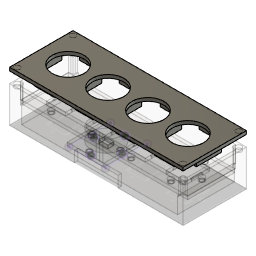
SW Full Enclosure (Autodesk Fusion 360 design; units mm, degrees)
Autodesk Fusion 360 part; units mm, degrees
sketch "Sketch1" plane through (0, 0, 0) normal (0, 1, 0) x (-1, 0, 0) in component "Button"
  arc A0 (78.25, -29) -> (80.25, -27) centre (78.25, -27) ccw
  line L0 (80.25, -27) -> (80.25, 27)
  arc A1 (80.25, 27) -> (78.25, 29) centre (78.25, 27) ccw
  line L1 (78.25, 29) -> (-78.25, 29)
  arc A2 (-78.25, 29) -> (-80.25, 27) centre (-78.25, 27) ccw
  line L2 (-80.25, 27) -> (-80.25, -27)
  arc A3 (-80.25, -27) -> (-78.25, -29) centre (-78.25, -27) ccw
  line L3 (-78.25, -29) -> (78.25, -29)
  circle A4 centre (-18.25, 0) radius 14.75
  circle A5 centre (18.25, 0) radius 14.75
  circle A6 centre (-54.75, 0) radius 14.75
  circle A7 centre (54.75, 0) radius 14.75
  line L4 (35, 19) -> (1.5, 19)
  line L5 (1.5, 19) -> (1.5, -19)
  line L6 (1.5, -19) -> (35, -19)
  line L7 (35, -19) -> (35, 19)
  line L8 (35, 19) -> (1.5, -19) construction
  line L9 (1.5, 19) -> (35, -19) construction
  point P0 (18.25, 0)
  dimension "d261" = 33.5
  dimension "d262" = 38
  dimension "d455" = 18.25
  constraint horizontal L4
  constraint perpendicular L4 L5
  constraint parallel L4 L6
  constraint parallel L5 L7
  constraint coincident L8 P0
  constraint coincident L9 P0
  measures "d261" distance of L5.end L6.end
  measures "d262" distance of L4.end L5.end
  measures "d455" distance of origin A5.centre
extrude "Extrude1" add sketch "Sketch1" along normal blind 3 contours A5 | L4 L5 L6 L7 makes body 1 in component "Button"
sketch "Sketch2" plane through (0, 3, 0) normal (0, 1, 0) x (-1, 0, 0) in component "Button"
  circle A0 centre (31.15, 0) radius 2.6
  line L0 (70, -19) -> (70, 19)
  line L1 (70, 19) -> (38, 19)
  line L2 (38, 19) -> (38, -19)
  line L3 (38, -19) -> (70, -19)
  line L4 (70, 19) -> (38, 19)
  line L5 (70, 19) -> (38, 19)
  line L6 (38, 19) -> (38, -19)
  line L7 (38, -19) -> (70, -19)
  line L8 (70, -19) -> (70, 19)
  line L9 (70, 19) -> (38, 19)
  line L10 (38, 19) -> (38, -19)
  line L11 (38, -19) -> (70, -19)
  circle A1 centre (31.15, 0) radius 2.6
  circle A2 centre (5.35, 0) radius 2.6
  line L12 (35, -19) -> (35, 19)
  line L13 (35, 19) -> (1.5, 19)
  line L14 (1.5, 19) -> (1.5, -19)
  line L15 (1.5, -19) -> (35, -19)
  circle A3 centre (18.25, -15.4) radius 2.6
  circle A4 centre (18.25, 15.4) radius 2.6
  line L16 (26.95, 11.2) -> (9.55, 11.2)
  line L17 (9.55, 11.2) -> (9.55, -11.2)
  line L18 (9.55, -11.2) -> (26.95, -11.2)
  line L19 (26.95, -11.2) -> (26.95, 11.2)
  line L20 (26.95, 11.2) -> (9.55, -11.2) construction
  line L21 (9.55, 11.2) -> (26.95, -11.2) construction
  line L22 (-1.75, 0) -> (-22.5, 0)
  line L23 (18.25, -15.4) -> (18.25, 15.4) construction
  line L24 (31.15, 0) -> (5.35, 0) construction
  point P0 (18.25, 0)
  point P1 (54.75, 0)
  point P2 (18.25, 0)
  point P3 (18.25, 0)
  dimension "d267" = 5.2
  dimension "d456" = 17.4
  dimension "d457" = 22.4
  dimension "d458" = 18.25
  dimension "d459" = 4.2
  dimension "d460" = 4.2
  constraint concentric A0 A1
  constraint equal A1 A4
  constraint equal A0 A2
  constraint equal A3 A4
  constraint horizontal L16
  constraint perpendicular L16 L17
  constraint parallel L16 L18
  constraint parallel L17 L19
  constraint coincident L20 P3
  constraint coincident L21 P3
  constraint coincident P3 L22
  constraint perpendicular L13 L23
  constraint perpendicular L23 L24
  constraint midpoint L23 P3
  constraint coincident P3 P2
  constraint midpoint L24 P3
  constraint coincident A2.centre L24.end
  constraint coincident A3.centre L23.start
  constraint coincident A4.centre L23.end
  constraint coincident A0.centre A1.centre
  constraint equal A2 A3
  measures "d267" diameter of A1
  measures "d456" distance of L17.end L18.end
  measures "d457" distance of L16.end L17.end
  measures "d458" distance of origin P3
  measures "d459" distance of L17 A2.centre
  measures "d460" distance of L18 A3.centre
extrude "Extrude2" cut sketch "Sketch2" along normal blind 2.4 from surface at -3 contours A0 A1 | A2 | A3 | A4 bodies 1 in component "Button"
sketch "Sketch3" plane through (0, 0, 0) normal (0, -1, 0) x (-1, 0, 0) in component "Button"
  circle A0 centre (18.25, -15.4) radius 1.9
  circle A1 centre (18.25, 15.4) radius 1.9
  circle A2 centre (31.15, 0) radius 2.6
  circle A3 centre (5.35, 0) radius 2.6
  circle A4 centre (18.25, 15.4) radius 2.6
  circle A5 centre (18.25, -15.4) radius 2.6
  line L0 (35, -19) -> (35, 19)
  line L1 (35, 19) -> (1.5, 19)
  line L2 (1.5, 19) -> (1.5, -19)
  line L3 (1.5, -19) -> (35, -19)
  circle A6 centre (31.15, 0) radius 1.9
  circle A7 centre (5.35, 0) radius 1.9
  point P0 (18.25, -15.4)
  point P1 (5.35, 0)
  point P2 (31.15, 0)
  point P3 (18.25, 15.4)
  dimension "d272" = 3.8
  dimension "d462" = 3.8
  constraint coincident P0 A0.centre
  constraint coincident P3 A1.centre
  constraint coincident P2 A2.centre
  constraint concentric A3 A7
  constraint equal A6 A7
  constraint equal A0 A7
  measures "d272" diameter of A1
  measures "d462" diameter of A6
extrude "Extrude7" cut sketch "Sketch3" against normal up to surface (3 mm away) contours A0 | A1 | A6 | A7 bodies 1 in component "Button"
sketch "Sketch4" plane through (0, 0, 0) normal (0, 1, 0) x (-1, 0, 0) in component "Button"
  line L0 (35, -19) -> (35, 19)
  line L1 (35, 19) -> (1.5, 19)
  line L2 (1.5, 19) -> (1.5, -19)
  line L3 (1.5, -19) -> (35, -19)
  line L4 (22.5, 2.75) -> (14, 2.75)
  line L5 (14, 2.75) -> (14, -2.75)
  line L6 (14, -2.75) -> (22.5, -2.75)
  line L7 (22.5, -2.75) -> (22.5, 2.75)
  line L8 (22.5, 2.75) -> (14, -2.75) construction
  line L9 (14, 2.75) -> (22.5, -2.75) construction
  line L10 (-1.75, 0) -> (-22.5, 0)
  point P0 (18.25, 0)
  dimension "d290" = 8.5
  dimension "d291" = 5.5
  dimension "d467" = 18.25
  constraint horizontal L4
  constraint perpendicular L4 L5
  constraint parallel L4 L6
  constraint parallel L5 L7
  constraint coincident L8 P0
  constraint coincident L9 P0
  constraint coincident P0 L10
  measures "d290" distance of L5.end L6.end
  measures "d291" distance of L4.end L5.end
  measures "d467" distance of origin P0
extrude "Extrude4" cut sketch "Sketch4" along normal up to surface (3 mm away) contours L4 L5 L6 L7 bodies 1 in component "Button"
sketch "Sketch5" plane through (0, 3, 0) normal (0, 1, 0) x (1, 0, 0) in component "Button"
  line L0 (-35, 19) -> (-35, -19)
  line L1 (-35, -19) -> (-1.5, -19)
  line L2 (-1.5, -19) -> (-1.5, 19)
  line L3 (-1.5, 19) -> (-35, 19)
  circle A0 centre (-18.25, -15.4) radius 1.9
  circle A1 centre (-5.35, 0) radius 1.9
  circle A2 centre (-31.15, 0) radius 1.9
  circle A3 centre (-18.25, 15.4) radius 1.9
  circle A4 centre (-18.25, 0) radius 14
  line L4 (-14, -2.75) -> (-22.5, -2.75)
  line L5 (-22.5, -2.75) -> (-22.5, 2.75)
  line L6 (-22.5, 2.75) -> (-14, 2.75)
  line L7 (-14, 2.75) -> (-14, -2.75)
  circle A5 centre (-18.25, -15.4) radius 1.9
  circle A6 centre (-5.35, 0) radius 1.9
  circle A7 centre (-31.15, 0) radius 1.9
  circle A8 centre (-18.25, 15.4) radius 1.9
  line L8 (-35, 19) -> (-35, -19)
  line L9 (-35, -19) -> (-1.5, -19)
  line L10 (-1.5, -19) -> (-1.5, 19)
  line L11 (-1.5, 19) -> (-35, 19)
  dimension "d465" = 18.25
  dimension "d466" = 28
  measures "d465" distance of origin A4.centre
  measures "d466" diameter of A4
extrude "Extrude5" add sketch "Sketch5" along normal blind 11 separate body contours A0 A4 A5 | A0 A1 A2 A3 A4 A5 A6 A7 A8 | A1 A4 A6 | A2 A4 A7 | A3 A4 A8 | L4 L5 L6 L7 picked at (-18.25, -13.8294) picked at (-5.1201, -0.5681) picked at (-31.2431, 0) picked at (-18.25, 13.8294) makes body 2 in component "Button"
sketch "Sketch6" plane through (0, 0, 0) normal (0, 1, 0) x (1, 0, 0) in component "Button"
  line L0 (-14.1, 2.65) -> (-22.4, 2.65)
  line L1 (-22.4, 2.65) -> (-22.4, -2.65)
  line L2 (-22.4, -2.65) -> (-14.1, -2.65)
  line L3 (-14.1, -2.65) -> (-14.1, 2.65)
  line L4 (-14.1, 2.65) -> (-22.4, -2.65) construction
  line L5 (-22.4, 2.65) -> (-14.1, -2.65) construction
  circle A0 centre (-18.25, 0) radius 14
  point P0 (-18.25, 0)
  dimension "d297" = 8.3
  dimension "d298" = 5.3
  constraint horizontal L0
  constraint perpendicular L0 L1
  constraint parallel L0 L2
  constraint parallel L1 L3
  constraint coincident L4 P0
  constraint coincident L5 P0
  constraint coincident P0 A0.centre
  measures "d297" distance of L1.end L2.end
  measures "d298" distance of L0.end L1.end
extrude "Extrude6" add sketch "Sketch6" along normal blind 7 contours L0 L1 L2 L3 bodies 2 in component "Button"
move_body "Move1" bodies 1 2 to x (1, 0, 0) y (0, 1, 0) z (0, 0, 1) at (-0.7, 0, 0) in component "Button"
move_body "Move2" bodies 2 1 to x (1, 0, 0) y (0, 1, 0) z (0, 0, 1) at (-0.9, 0, 0) in component "Button"
sketch "Sketch1 (2)" plane through (0, 0, 0) normal (0, 1, 0) x (1, 0, 0) in component "Button Base (1)"
  line L0 (76.05, -21.5) -> (0, -21.5)
  line L1 (0, -21.5) -> (0, 21.5)
  line L2 (0, 21.5) -> (76.05, 21.5)
  line L3 (76.05, 21.5) -> (76.05, -21.5)
  line L4 (76.05, -21.5) -> (0, 21.5) construction
  line L5 (0, -21.5) -> (76.05, 21.5) construction
  line L6 (1.75, 0) -> (22.5, 0)
  point P0 (38.025, 0)
  dimension "d337" = 76.05
  dimension "d338" = 43
  constraint horizontal L0
  constraint perpendicular L0 L1
  constraint parallel L0 L2
  constraint parallel L1 L3
  constraint coincident L4 P0
  constraint coincident L5 P0
  constraint coincident P0 L6
  constraint coincident origin L1
  measures "d337" distance of L1.end L2.end
  measures "d338" distance of L0.start L2.end
extrude "Extrude1'" add sketch "Sketch1 (2)" along normal blind 3 separate body makes body 3 in component "Button Base (1)"
sketch "Sketch2 (2)" plane through (0, 3, 0) normal (0, 1, 0) x (-1, 0, 0) in component "Button Base (1)"
  line L0 (-76.05, -21.5) -> (0, -21.5)
  line L1 (0, -21.5) -> (0, 21.5)
  line L2 (0, 21.5) -> (-76.05, 21.5)
  line L3 (-76.05, 21.5) -> (-76.05, -21.5)
  line L4 (-9.55, -11.2) -> (-26.95, -11.2)
  line L5 (-26.95, -11.2) -> (-26.95, 11.2)
  line L6 (-26.95, 11.2) -> (-9.55, 11.2)
  line L7 (-9.55, 11.2) -> (-9.55, -11.2)
  line L8 (-9.55, -11.2) -> (-26.95, 11.2) construction
  line L9 (-26.95, -11.2) -> (-9.55, 11.2) construction
  line L10 (-1.75, 0) -> (-22.5, 0)
  point P0 (-18.25, 0)
  dimension "d341" = 17.4
  dimension "d342" = 22.4
  dimension "d343" = 18.25
  constraint horizontal L4
  constraint perpendicular L4 L5
  constraint parallel L4 L6
  constraint parallel L5 L7
  constraint coincident L8 P0
  constraint coincident L9 P0
  constraint coincident P0 L10
  measures "d341" distance of L5.end L6.end
  measures "d342" distance of L4.end L5.end
  measures "d343" distance of origin P0
extrude "Extrude2'" cut sketch "Sketch2 (2)" against normal up to surface (3 mm away) contours L4 L5 L6 L7 bodies 3 in component "Button Base (1)"
sketch "Sketch3 (2)" plane through (0, 3, 0) normal (0, 1, 0) x (-1, 0, 0) in component "Button Base (1)"
  line L0 (-9.55, 11.2) -> (-9.55, -11.2)
  line L1 (-9.55, -11.2) -> (-26.95, -11.2)
  line L2 (-26.95, -11.2) -> (-26.95, 11.2)
  line L3 (-26.95, 11.2) -> (-9.55, 11.2)
  line L4 (-76.05, -21.5) -> (0, -21.5)
  line L5 (0, -21.5) -> (0, 21.5)
  line L6 (0, 21.5) -> (-76.05, 21.5)
  line L7 (-76.05, 21.5) -> (-76.05, -21.5)
  circle A0 centre (-5.35, 0) radius 2.6
  circle A1 centre (-18.25, -15.4) radius 2.6
  circle A2 centre (-31.15, 0) radius 2.6
  circle A3 centre (-18.25, 15.4) radius 2.6
  line L8 (-18.25, 15.4) -> (-18.25, -15.4) construction
  line L9 (-1.75, 0) -> (-22.5, 0)
  point P0 (-18.25, -11.2)
  dimension "d346" = 5.2
  dimension "d347" = 4.2
  dimension "d348" = 4.2
  dimension "d349" = 4.2
  dimension "d350" = 4.2
  constraint equal A1 A2
  constraint equal A2 A3
  constraint equal A0 A3
  constraint midpoint L1 P0
  constraint perpendicular L1 L8
  constraint coincident A3.centre L8
  constraint coincident A3.centre L8.start
  constraint coincident P0 L8
  constraint coincident A1.centre L8
  constraint coincident A1.centre L8.end
  constraint coincident A2.centre L9
  constraint coincident A0.centre L9
  measures "d346" diameter of A1
  measures "d347" distance of L3 A3.centre
  measures "d348" distance of L1 A1.centre
  measures "d349" distance of L0 A0.centre
  measures "d350" distance of L2 A2.centre
extrude "Extrude3" cut sketch "Sketch3 (2)" against normal blind 2.4 contours A0 L9 | A0 L9 | A1 | A2 | A3 bodies 3 in component "Button Base (1)"
sketch "Sketch4 (2)" plane through (0, 3, 0) normal (0, 1, 0) x (-1, 0, 0) in component "Button Base (1)"
  circle A0 centre (-18.25, -15.4) radius 2.6
  circle A1 centre (-31.15, 0) radius 2.6
  circle A2 centre (-5.35, 0) radius 2.6
  circle A3 centre (-18.25, 15.4) radius 2.6
  line L0 (-9.55, 11.2) -> (-9.55, -11.2)
  line L1 (-9.55, -11.2) -> (-26.95, -11.2)
  line L2 (-26.95, -11.2) -> (-26.95, 11.2)
  line L3 (-26.95, 11.2) -> (-9.55, 11.2)
  line L4 (-76.05, -21.5) -> (0, -21.5)
  line L5 (0, -21.5) -> (0, 21.5)
  line L6 (0, 21.5) -> (-76.05, 21.5)
  line L7 (-76.05, 21.5) -> (-76.05, -21.5)
  circle A4 centre (-18.25, -15.4) radius 1.9
  circle A5 centre (-31.15, 0) radius 1.9
  circle A6 centre (-18.25, 15.4) radius 1.9
  circle A7 centre (-5.35, 0) radius 1.9
  dimension "d353" = 3.8
  constraint concentric A0 A4
  constraint concentric A1 A5
  constraint concentric A3 A6
  constraint concentric A2 A7
  constraint equal A4 A7
  constraint equal A5 A6
  constraint equal A6 A7
  measures "d353" diameter of A7
extrude "Extrude4'" cut sketch "Sketch4 (2)" against normal up to surface (3 mm away) contours A4 | A5 | A6 | A7 bodies 3 in component "Button Base (1)"
sketch "Sketch5 (2)" plane through (0, 0, 21.5) normal (0, 0, 1) x (1, 0, 0) in component "Button Base (1)"
  line L0 (0, 0) -> (76.05, 0)
  line L1 (76.05, 0) -> (76.05, 3)
  line L2 (76.05, 3) -> (0, 3)
  line L3 (0, 3) -> (0, 0)
  line L4 (18.25, 5) -> (18.25, -2) construction
  line L5 (26.95, 0) -> (9.55, 0) construction
  line L6 (9.55, 0) -> (9.55, 3)
  line L7 (9.55, 3) -> (26.95, 3) construction
  line L8 (26.95, 3) -> (26.95, 0) construction
  line L9 (26.95, 0) -> (9.55, 3) construction
  line L10 (9.55, 0) -> (26.95, 3) construction
  line L11 (9.55, 0) -> (11.05, 1.5)
  line L12 (9.55, 0) -> (12.4248, 0) construction
  line L13 (9.55, 3) -> (9.55, 1.5) construction
  line L14 (9.55, 1.5) -> (11.05, 1.5)
  line L15 (9.55, 1.5) -> (9.55, 0) construction
  line L16 (26.95, 0) -> (26.95, 1.5)
  line L17 (26.95, 1.5) -> (25.45, 1.5)
  line L18 (25.45, 1.5) -> (26.95, 0)
  point P0 (18.25, 1.5)
  dimension "d358" = 18.25
  dimension "d359" = 17.4
  dimension "d360" = 3
  dimension "d361" = 45
  dimension "d362" = 1.5
  dimension "d363" = 1.5
  dimension "d364" = 1.5
  dimension "d365" = 1.5
  constraint vertical L4
  constraint horizontal L5
  constraint perpendicular L5 L6
  constraint parallel L5 L7
  constraint parallel L6 L8
  constraint coincident L9 P0
  constraint coincident L10 P0
  constraint midpoint L4 P0
  constraint horizontal L12
  constraint coincident L6 L13.end
  constraint perpendicular L6 L14
  constraint coincident L11.end L14.end
  constraint perpendicular L5 L16
  constraint perpendicular L8 L17
  measures "d358" distance of L0.start L4
  measures "d359" distance of L6.end L7.end
  measures "d360" distance of L5.end L6.end
  measures "d361" angle of L11 L12
  measures "d362" distance of L6.end L13.end
  measures "d363" distance of L0 P0
  measures "d364" distance of L5.start L16.end
  measures "d365" distance of L16.end L17.end
extrude "Extrude5'" add sketch "Sketch5 (2)" along normal mid plane 10 from surface at -21.5 contours L16 L17 L18 | L6 L11 L14 bodies 3 in component "Button Base (1)"
pattern_path "PathPattern1" count 2 spacing 36.5 from (0, 3, -21.5) along 1 edges at (38.025, 3, -21.5) of "Extrude2'", "Extrude3", "Extrude4'", "Extrude5'" on bodies 3 in component "Button Base (1)"
mirror "Mirror1" about plane through (0, 0, 0) normal (1, 0, 0) of bodies 3 makes body 4 in component "Button Base (1)"
combine "Combine1" operation add target body 3 tool bodies 4 in component "Button Base (1)"
sketch "Sketch1 (3)" plane through (0, 0, 0) normal (0, 1, 0) x (1, 0, 0) in component "Button Box (1)"
  line L0 (79.25, -29) -> (0, -29)
  line L1 (0, -29) -> (0, 29)
  line L2 (0, 29) -> (79.25, 29)
  line L3 (79.25, 29) -> (79.25, -29)
  line L4 (79.25, -29) -> (0, 29) construction
  line L5 (0, -29) -> (79.25, 29) construction
  line L6 (1.75, 0) -> (22.5, 0)
  point P0 (39.625, 0)
  dimension "d372" = 79.25
  dimension "d379" = 58
  constraint horizontal L0
  constraint perpendicular L0 L1
  constraint parallel L0 L2
  constraint parallel L1 L3
  constraint coincident L4 P0
  constraint coincident L5 P0
  constraint coincident P0 L6
  constraint coincident origin L1
  measures "d372" distance of L1.end L2.end
  measures "d379" distance of L0.start L2.end
extrude "Extrude1''" add sketch "Sketch1 (3)" along normal blind 33 separate body makes body 5 in component "Button Box (1)"
shell "Shell1" thickness 3 removed faces 1 at (52.8333, 33, 9.6667) on bodies 5 in component "Button Box (1)"
sketch "Sketch2 (3)" plane through (0, 33, 0) normal (0, 1, 0) x (-1, 0, 0) in component "Button Box (1)"
  line L0 (-76.25, -26) -> (-76.25, 26)
  line L1 (-76.25, 26) -> (-3, 26)
  line L2 (-3, 26) -> (-3, -26)
  line L3 (-3, -26) -> (-76.25, -26)
  line L4 (-79.25, -29) -> (0, -29)
  line L5 (0, -29) -> (0, 29)
  line L6 (0, 29) -> (-79.25, 29)
  line L7 (-79.25, 29) -> (-79.25, -29)
  line L8 (-76.25, 26) -> (-71.25, 26)
  line L9 (-71.25, 26) -> (-71.25, -26)
  line L10 (-71.25, -26) -> (-76.25, -26)
  line L11 (-76.25, -26) -> (-76.25, 26)
  line L12 (-76.25, 26) -> (-71.25, -26) construction
  line L13 (-71.25, 26) -> (-76.25, -26) construction
  point P0 (-73.75, 0)
  dimension "d378" = 52
  dimension "d380" = 5
  dimension "d382" = 73.75
  constraint horizontal L8
  constraint perpendicular L8 L9
  constraint parallel L8 L10
  constraint parallel L9 L11
  constraint coincident L1 L0.end
  constraint coincident L12 P0
  constraint coincident L13 P0
  measures "d378" distance of L0.end L0.start
  measures "d380" distance of L9.end L0.start
  measures "d382" distance of origin P0
extrude "Extrude2''" add sketch "Sketch2 (3)" along normal blind 18 from surface at -33 contours L0 L1 L3 L8 L9 L10 L11 bodies 5 in component "Button Box (1)"
sketch "Sketch3 (3)" plane through (0, 33, 0) normal (0, 1, 0) x (-1, 0, 0) in component "Button Box (1)"
  line L0 (-76.25, -26) -> (-76.25, 26)
  line L1 (-76.25, 26) -> (-3, 26)
  line L2 (-3, 26) -> (-3, -26)
  line L3 (-3, -26) -> (-76.25, -26)
  line L4 (-79.25, -29) -> (0, -29)
  line L5 (0, -29) -> (0, 29)
  line L6 (0, 29) -> (-79.25, 29)
  line L7 (-79.25, 29) -> (-79.25, -29)
  line L8 (-79.25, -29) -> (-72.25, -29)
  line L9 (-72.25, -29) -> (-72.25, -22)
  line L10 (-72.25, -22) -> (-79.25, -22)
  line L11 (-79.25, -22) -> (-79.25, -29)
  line L12 (-79.25, 29) -> (-72.25, 29)
  line L13 (-72.25, 29) -> (-72.25, 22)
  line L14 (-72.25, 22) -> (-79.25, 22)
  line L15 (-79.25, 22) -> (-79.25, 29)
  dimension "d386" = 7
  dimension "d387" = 7
  dimension "d388" = 7
  dimension "d389" = 7
  constraint horizontal L8
  constraint vertical L9
  constraint horizontal L10
  constraint vertical L11
  constraint coincident L4.start L7.end
  constraint horizontal L12
  constraint vertical L13
  constraint horizontal L14
  constraint vertical L15
  constraint coincident L6.end L7.start
  measures "d386" distance of L4.start L8.end
  measures "d387" distance of L4.start L10.end
  measures "d388" distance of L6.end L12.end
  measures "d389" distance of L6.end L14.end
extrude "Extrude3'" add sketch "Sketch3 (3)" along normal up to near side of body 5 contours L0 L3 L9 L10 | L0 L1 L13 L14 bodies 5 in component "Button Box (1)"
sketch "Sketch4 (3)" plane through (0, 33, 0) normal (0, 1, 0) x (-1, 0, 0) in component "Button Box (1)"
  line L0 (-76.25, -22) -> (-76.25, 22)
  line L1 (-76.25, 22) -> (-72.25, 22)
  line L2 (-72.25, 22) -> (-72.25, 26)
  line L3 (-72.25, 26) -> (-3, 26)
  line L4 (-3, 26) -> (-3, -26)
  line L5 (-3, -26) -> (-72.25, -26)
  line L6 (-72.25, -26) -> (-72.25, -22)
  line L7 (-72.25, -22) -> (-76.25, -22)
  line L8 (-79.25, -29) -> (0, -29)
  line L9 (0, -29) -> (0, 29)
  line L10 (0, 29) -> (-79.25, 29)
  line L11 (-79.25, 29) -> (-79.25, -29)
  circle A0 centre (-75.75, 25.5) radius 2.6
  circle A1 centre (-75.75, -25.5) radius 2.6
  dimension "d393" = 3.5
  dimension "d394" = 3.5
  dimension "d397" = 3.5
  dimension "d398" = 3.5
  dimension "d399" = 5.2
  constraint equal A0 A1
  measures "d393" distance of L11 A0.centre
  measures "d394" distance of L10 A0.centre
  measures "d397" distance of L8 A1.centre
  measures "d398" distance of L11 A1.centre
  measures "d399" diameter of A1
extrude "Extrude4''" cut sketch "Sketch4 (3)" against normal blind 2.4 contours A0 | A1 bodies 5 in component "Button Box (1)"
fillet "Fillet1" radius 2 2 edges at (72.25, 25.5, 22) (72.25, 25.5, -22) on bodies 5 in component "Button Box (1)"
sketch "Sketch5 (3)" plane through (0, 33, 0) normal (0, 1, 0) x (-1, 0, 0) in component "Button Box (1)"
  arc A0 (-72.25, -24) -> (-74.25, -22) centre (-74.25, -24) ccw
  line L0 (-74.25, -22) -> (-76.25, -22)
  line L1 (-76.25, -22) -> (-76.25, 22)
  line L2 (-76.25, 22) -> (-74.25, 22)
  arc A1 (-74.25, 22) -> (-72.25, 24) centre (-74.25, 24) ccw
  line L3 (-72.25, 24) -> (-72.25, 26)
  line L4 (-72.25, 26) -> (-3, 26)
  line L5 (-3, 26) -> (-3, -26)
  line L6 (-3, -26) -> (-72.25, -26)
  line L7 (-72.25, -26) -> (-72.25, -24)
  circle A2 centre (-75.75, -25.5) radius 2.6
  circle A3 centre (-75.75, 25.5) radius 2.6
  line L8 (-79.25, -29) -> (0, -29)
  line L9 (0, -29) -> (0, 29)
  line L10 (0, 29) -> (-79.25, 29)
  line L11 (-79.25, 29) -> (-79.25, -29)
  line L12 (-3, -26) -> (0, -26)
  line L13 (0, 26) -> (-3, 26)
  constraint coincident L5.end L6.start
  constraint coincident L9 L12.end
  constraint perpendicular L9 L12
  constraint coincident L9 L13.start
  constraint coincident L4.end L5.start
  constraint perpendicular L5 L13
extrude "Extrude5''" cut sketch "Sketch5 (3)" against normal up to surface (30 mm away) contours L5 L9 L12 L13 bodies 5 in component "Button Box (1)"
sketch "Sketch6 (2)" plane through (0, 0, 29) normal (0, 0, 1) x (1, 0, 0) in component "Button Box (1)"
  line L0 (0, 0) -> (79.25, 0)
  line L1 (79.25, 0) -> (79.25, 33)
  line L2 (79.25, 33) -> (0, 33)
  line L3 (0, 33) -> (0, 0)
  line L4 (0, 0) -> (20, 0)
  line L5 (20, 0) -> (20, 10)
  line L6 (20, 10) -> (0, 10)
  line L7 (0, 10) -> (0, 0)
  dimension "d405" = 20
  dimension "d406" = 10
  constraint horizontal L4
  constraint vertical L5
  constraint horizontal L6
  constraint vertical L7
  constraint coincident L0.start L3.end
  measures "d405" distance of L0.start L4.end
  measures "d406" distance of L0.start L6.end
extrude "Extrude6'" cut sketch "Sketch6 (2)" against normal blind 3 contours L0 L3 L4 L5 L6 L7 bodies 5 in component "Button Box (1)"
mirror "Mirror1'" about plane through (0, 0, 0) normal (1, 0, 0) of bodies 5 makes body 6 in component "Button Box (1)"
combine "Combine1'" operation add target body 6 tool bodies 5 in component "Button Box (1)"
sketch "Sketch1 (4)" plane through (0, 3, 0) normal (0, 1, 0) x (-1, 0, 0) in component "Button Box Lid (1)"
  line L0 (9.55, -11.2) -> (9.55, 11.2)
  line L1 (9.55, 11.2) -> (26.95, 11.2)
  line L2 (26.95, 11.2) -> (26.95, -11.2)
  line L3 (26.95, -11.2) -> (9.55, -11.2)
  circle A0 centre (18.25, 15.4) radius 2.6
  circle A1 centre (5.35, 0) radius 2.6
  circle A2 centre (31.15, 0) radius 2.6
  circle A3 centre (18.25, -15.4) radius 2.6
  line L4 (46.05, -11.2) -> (46.05, 11.2)
  line L5 (46.05, 11.2) -> (63.45, 11.2)
  line L6 (63.45, 11.2) -> (63.45, -11.2)
  line L7 (63.45, -11.2) -> (46.05, -11.2)
  circle A4 centre (67.65, 0) radius 2.6
  circle A5 centre (41.85, 0) radius 2.6
  circle A6 centre (54.75, -15.4) radius 2.6
  circle A7 centre (54.75, 15.4) radius 2.6
  circle A8 centre (-54.75, 15.4) radius 2.6
  circle A9 centre (-54.75, -15.4) radius 2.6
  circle A10 centre (-41.85, 0) radius 2.6
  circle A11 centre (-67.65, 0) radius 2.6
  line L8 (-46.05, 11.2) -> (-46.05, -11.2)
  line L9 (-46.05, -11.2) -> (-63.45, -11.2)
  line L10 (-63.45, -11.2) -> (-63.45, 11.2)
  line L11 (-63.45, 11.2) -> (-46.05, 11.2)
  circle A12 centre (-18.25, -15.4) radius 2.6
  circle A13 centre (-31.15, 0) radius 2.6
  circle A14 centre (-5.35, 0) radius 2.6
  circle A15 centre (-18.25, 15.4) radius 2.6
  line L12 (-9.55, 11.2) -> (-9.55, -11.2)
  line L13 (-9.55, -11.2) -> (-26.95, -11.2)
  line L14 (-26.95, -11.2) -> (-26.95, 11.2)
  line L15 (-26.95, 11.2) -> (-9.55, 11.2)
  line L16 (-76.05, -21.5) -> (76.05, -21.5)
  line L17 (76.05, -21.5) -> (76.05, 21.5)
  line L18 (76.05, 21.5) -> (-76.05, 21.5)
  line L19 (-76.05, 21.5) -> (-76.05, -21.5)
  line L20 (-1.75, 0) -> (-22.5, 0)
  line L21 (-79.25, 29) -> (0, 29)
  line L22 (0, 29) -> (0, -29)
  line L23 (0, -29) -> (-79.25, -29)
  line L24 (-79.25, -29) -> (-79.25, 29)
  line L25 (-79.25, 29) -> (0, -29) construction
  line L26 (0, 29) -> (-79.25, -29) construction
  point P0 (-39.625, 0)
  dimension "d413" = 79.25
  dimension "d414" = 58
  constraint horizontal L21
  constraint perpendicular L21 L22
  constraint parallel L21 L23
  constraint parallel L22 L24
  constraint coincident L25 P0
  constraint coincident L26 P0
  constraint coincident L20 P0
  constraint coincident origin L22
  measures "d413" distance of L22.end L23.end
  measures "d414" distance of L21.start L23.end
extrude "Extrude1'''" add sketch "Sketch1 (4)" along normal blind 3 separate body contours A8 | A9 | A10 | A11 | L8 L9 L10 L11 | A12 | A13 | A14 L20 | A14 L20 | A15 | L12 L13 L14 L15 | L16 L18 L19 L22 | L16 L18 L19 L21 L22 L23 L24 makes body 7 in component "Button Box Lid (1)"
sketch "Sketch2 (4)" plane through (0, 6, 0) normal (0, 1, 0) x (-1, 0, 0) in component "Button Box Lid (1)"
  line L0 (-79.25, -29) -> (0, -29)
  line L1 (0, -29) -> (0, 29)
  line L2 (0, 29) -> (-79.25, 29)
  line L3 (-79.25, 29) -> (-79.25, -29)
  circle A0 centre (-18.25, 0) radius 14.5
  line L4 (-1.75, 0) -> (-22.5, 0)
  circle A1 centre (-54.75, 0) radius 14.5
  dimension "d417" = 29
  dimension "d418" = 18.25
  dimension "d419" = 36.5
  constraint coincident A0.centre L4
  constraint equal A0 A1
  constraint coincident L4 A1.centre
  measures "d417" diameter of A0
  measures "d418" distance of origin A0.centre
  measures "d419" distance of A0.centre A1.centre
extrude "Extrude2'''" cut sketch "Sketch2 (4)" against normal up to surface (3 mm away) contours A0 | A1 bodies 7 in component "Button Box Lid (1)"
sketch "Sketch3 (4)" plane through (0, 3, 0) normal (0, 1, 0) x (-1, 0, 0) in component "Button Box Lid (1)"
  circle A0 centre (-75.75, -25.5) radius 2.6
  circle A1 centre (-75.75, 25.5) radius 2.6
  line L0 (-79.25, -29) -> (-79.25, 29)
  line L1 (-79.25, 29) -> (0, 29)
  line L2 (0, -29) -> (-79.25, -29)
  dimension "d422" = 5.2
  dimension "d423" = 3.5
  dimension "d424" = 3.5
  dimension "d425" = 3.5
  dimension "d426" = 3.5
  constraint equal A0 A1
  measures "d422" diameter of A1
  measures "d423" distance of A1.centre L0
  measures "d424" distance of A1.centre L1
  measures "d425" distance of A0.centre L0
  measures "d426" distance of A0.centre L2
extrude "Extrude3''" cut sketch "Sketch3 (4)" along normal blind 2.4 bodies 7 in component "Button Box Lid (1)"
sketch "Sketch4 (4)" plane through (0, 3, 0) normal (0, -1, 0) x (1, 0, 0) in component "Button Box Lid (1)"
  circle A0 centre (75.75, -25.5) radius 2.6
  circle A1 centre (75.75, 25.5) radius 2.6
  circle A2 centre (18.25, 0) radius 14.5
  circle A3 centre (54.75, 0) radius 14.5
  line L0 (0, -29) -> (79.25, -29)
  line L1 (79.25, -29) -> (79.25, 29)
  line L2 (79.25, 29) -> (0, 29)
  line L3 (0, 29) -> (0, -29)
  line L4 (72, -19.5) -> (37.5, -19.5)
  line L5 (37.5, -19.5) -> (37.5, 19.5)
  line L6 (37.5, 19.5) -> (72, 19.5)
  line L7 (72, 19.5) -> (72, -19.5)
  line L8 (72, -19.5) -> (37.5, 19.5) construction
  line L9 (37.5, -19.5) -> (72, 19.5) construction
  line L10 (35.5, 21.5) -> (74, 21.5)
  line L11 (74, 21.5) -> (74, -21.5)
  line L12 (74, -21.5) -> (35.5, -21.5)
  line L13 (35.5, -19.5) -> (35.5, 19.5)
  line L14 (35.5, 21.5) -> (74, -21.5) construction
  line L15 (74, 21.5) -> (35.5, -21.5) construction
  line L16 (1, 19.5) -> (35.5, 19.5)
  line L17 (35.5, 19.5) -> (35.5, -19.5)
  line L18 (35.5, -19.5) -> (1, -19.5)
  line L19 (1, -19.5) -> (1, 19.5)
  line L20 (1, 19.5) -> (35.5, -19.5) construction
  line L21 (35.5, 19.5) -> (1, -19.5) construction
  line L22 (35.5, -21.5) -> (0, -21.5)
  line L23 (35.5, 21.5) -> (0, 21.5)
  line L24 (0, -21.5) -> (0, 21.5)
  line L25 (74, -21.5) -> (72, -21.5)
  line L26 (72, -19.5) -> (72, -11.5)
  line L27 (72, -11.5) -> (74, -11.5)
  line L28 (74, -11.5) -> (74, -21.5)
  line L29 (74, -21.5) -> (64, -21.5)
  line L30 (64, -21.5) -> (64, -19.5)
  line L31 (64, -19.5) -> (72.2093, -19.5)
  line L32 (74, -19.5) -> (74, -21.5)
  line L33 (74, 21.5) -> (72, 21.5)
  line L34 (72, 19.5) -> (72, 11.5)
  line L35 (72, 11.5) -> (74, 11.5)
  line L36 (74, 11.5) -> (74, 21.5)
  line L37 (74, 21.5) -> (64, 21.5)
  line L38 (64, 19.5) -> (72.2093, 19.5)
  line L39 (74, 19.5) -> (74, 21.5)
  line L40 (64, 19.5) -> (64, 21.5)
  line L41 (37.5, 19.5) -> (27.5, 19.5)
  line L42 (27.5, 19.5) -> (27.5, 21.5)
  line L43 (27.5, 21.5) -> (37.5, 21.5)
  line L44 (35.5, 19.5) -> (45.5, 19.5)
  line L45 (45.5, 19.5) -> (45.5, 21.5)
  line L46 (45.5, 21.5) -> (35.5, 21.5)
  line L47 (35.5, 21.5) -> (35.5, 19.5)
  line L48 (37.5, 21.5) -> (35.5, 21.5)
  line L49 (35.5, 19.5) -> (35.5, 11.5)
  line L50 (35.5, 11.5) -> (37.5, 11.5)
  line L51 (37.5, 11.5) -> (37.5, 21.5)
  line L52 (37.5, -19.5) -> (27.5, -19.5)
  line L53 (27.5, -19.5) -> (27.5, -21.5)
  line L54 (27.5, -21.5) -> (37.5, -21.5)
  line L55 (35.5, -19.5) -> (45.5, -19.5)
  line L56 (45.5, -19.5) -> (45.5, -21.5)
  line L57 (45.5, -21.5) -> (35.5, -21.5)
  line L58 (37.5, -21.5) -> (35.5, -21.5)
  line L59 (35.5, -21.5) -> (35.5, -11.5)
  line L60 (35.5, -11.5) -> (37.5, -11.5)
  line L61 (37.5, -11.5) -> (37.5, -21.5)
  line L62 (0, -21.5) -> (10, -21.5)
  line L63 (10, -21.5) -> (10, -19.5)
  line L64 (10, -19.5) -> (1, -19.5)
  line L65 (0, -19.5) -> (0, -21.5)
  line L66 (0, 21.5) -> (1, 21.5)
  line L67 (1, 19.5) -> (1, 11.5)
  line L68 (1, 11.5) -> (0, 11.5)
  line L69 (0, 11.5) -> (0, 21.5)
  line L70 (0, 21.5) -> (10, 21.5)
  line L71 (10, 21.5) -> (10, 19.5)
  line L72 (10, 19.5) -> (1, 19.5)
  line L73 (0, 19.5) -> (0, 21.5)
  line L74 (0, -21.5) -> (1, -21.5)
  line L75 (1, -19.5) -> (1, -11.5)
  line L76 (1, -11.5) -> (0, -11.5)
  line L77 (0, -11.5) -> (0, -21.5)
  point P0 (54.75, 0)
  point P1 (54.75, 0)
  point P2 (18.25, 0)
  dimension "d429" = 34.5
  dimension "d430" = 39
  dimension "d431" = 2
  dimension "d432" = 2
  dimension "d433" = 34.5
  dimension "d434" = 39
  dimension "d435" = 2
  dimension "d436" = 10
  dimension "d437" = 10
  dimension "d438" = 10
  dimension "d439" = 10
  dimension "d440" = 10
  dimension "d441" = 10
  dimension "d442" = 2
  dimension "d443" = 10
  dimension "d444" = 10
  dimension "d445" = 2
  dimension "d446" = 10
  dimension "d447" = 10
  dimension "d448" = 10
  dimension "d449" = 10
  dimension "d450" = 10
  dimension "d451" = 10
  constraint horizontal L4
  constraint perpendicular L4 L5
  constraint parallel L4 L6
  constraint parallel L5 L7
  constraint coincident L8 P1
  constraint coincident L9 P1
  constraint coincident P1 P0
  constraint horizontal L10
  constraint perpendicular L10 L11
  constraint parallel L10 L12
  constraint parallel L11 L13
  constraint coincident L14 P1
  constraint coincident L15 P1
  constraint horizontal L16
  constraint perpendicular L16 L17
  constraint parallel L16 L18
  constraint parallel L17 L19
  constraint coincident L20 P2
  constraint coincident L21 P2
  constraint coincident P2 A2.centre
  constraint coincident L3 L22.end
  constraint perpendicular L3 L22
  constraint coincident L3 L23.end
  constraint perpendicular L3 L23
  constraint horizontal L25
  constraint vertical L26
  constraint horizontal L27
  constraint vertical L28
  constraint horizontal L29
  constraint vertical L30
  constraint horizontal L31
  constraint vertical L32
  constraint coincident L14 L31.end
  constraint horizontal L33
  constraint vertical L34
  constraint horizontal L35
  constraint vertical L36
  constraint horizontal L37
  constraint horizontal L38
  constraint vertical L39
  constraint coincident L15 L38.end
  constraint perpendicular L37 L40
  constraint coincident L6 L38.end
  constraint coincident L4 L30.end
  constraint horizontal L41
  constraint vertical L42
  constraint horizontal L43
  constraint horizontal L44
  constraint vertical L45
  constraint horizontal L46
  constraint vertical L47
  constraint horizontal L48
  constraint vertical L49
  constraint horizontal L50
  constraint vertical L51
  constraint horizontal L52
  constraint vertical L53
  constraint horizontal L54
  constraint horizontal L55
  constraint vertical L56
  constraint horizontal L57
  constraint horizontal L58
  constraint vertical L59
  constraint horizontal L60
  constraint vertical L61
  constraint horizontal L62
  constraint vertical L63
  constraint horizontal L64
  constraint vertical L65
  constraint horizontal L66
  constraint vertical L67
  constraint horizontal L68
  constraint vertical L69
  constraint horizontal L70
  constraint vertical L71
  constraint horizontal L72
  constraint vertical L73
  constraint horizontal L74
  constraint vertical L75
  constraint horizontal L76
  constraint vertical L77
  measures "d429" distance of L5.end L6.end
  measures "d430" distance of L4.end L5.end
  measures "d431" distance of L4 L12
  measures "d432" distance of L7 L11
  measures "d433" distance of L13.start L18.end
  measures "d434" distance of L16.start L18.end
  measures "d435" distance of L16 L23
  measures "d436" distance of L11.end L27.end
  measures "d437" distance of L11.end L29.end
  measures "d438" distance of L10.end L35.end
  measures "d439" distance of L10.end L37.end
  measures "d440" distance of L5.end L41.end
  measures "d441" distance of L13.end L44.end
  measures "d442" distance of L43.end L10.start
  measures "d443" distance of L43.end L50.end
  measures "d444" distance of L4.end L52.end
  measures "d445" distance of L4.end L54.end
  measures "d446" distance of L13.start L55.end
  measures "d447" distance of L54.end L60.end
  measures "d448" distance of L22.end L62.end
  measures "d449" distance of L23.end L68.end
  measures "d450" distance of L23.end L70.end
  measures "d451" distance of L22.end L76.end
extrude "Extrude4'''" add sketch "Sketch4 (4)" along normal blind 8 contours L3 L19 L24 L68 L76 | L18 L22 L53 L63 | L16 L23 L42 L71 | L4 L12 L30 L56 | L5 L13 L17 L50 L60 | L6 L10 L40 L45 | L7 L11 L27 L35 bodies 7 in component "Button Box Lid (1)"
mirror "Mirror1''" about plane through (0, 0, 0) normal (1, 0, 0) of bodies 7 makes body 8 in component "Button Box Lid (1)"
combine "Combine1''" operation add target body 7 tool bodies 8 in component "Button Box Lid (1)"
move_body "Move1'" bodies 3 to x (1, 0, 0) y (0, 1, 0) z (0, 0, 1) at (0, 15, 0) in component "Button Base (1)"
component "Button" placed x (1, 0, 0) y (0, 1, 0) z (0, 0, 1) at (0, 0, 0)
component "Button Base (1)" placed x (1, 0, 0) y (0, 1, 0) z (0, 0, 1) at (0, 0, 0)
component "Button Box (1)" placed x (1, 0, 0) y (0, 1, 0) z (0, 0, 1) at (0, 0, 0)
component "Button Box Lid (1)" placed x (1, 0, 0) y (0, 1, 0) z (0, 0, 1) at (0, 0, 0)
component "Component'" placed x (1, 0, 0) y (0, 1, 0) z (0, 0, 1) at (0, 0, 0)
component "Component" placed x (1, 0, 0) y (0, 1, 0) z (0, 0, 1) at (0, 0, 0) in component "Button Box Lid (1)"
equation "boxLength = 160.5 mm"
equation "boxWidth = 58 mm"
equation "boxHeight = 33 mm"
equation "wallThickness = 3 mm"
equation "BaseLength = 152.8 mm"
equation "BaseWidth = 43 mm"
equation "BaseThickness = 4 mm"
equation "capsenseLength = 22.4 mm"
equation "capsenseWidth = 17.4 mm"
equation "capsenseDFE = 10.4 mm"
equation "capsenseDFCE = 18.80 mm"
equation "magnetOD = 5.2 mm"
equation "magnetDepth = 2.4 mm"
equation "magnetDFCapsense = 4.2 mm"
equation "BaseWallThickness = 2 mm"
equation "BaseWallHeight = 8 mm"
equation "CapsenseThick = 1.5 mm"
equation "MagnetThruHoleOD = 3.8 mm"
equation "BaseWallSpacing = 11 mm"
equation "PressFitTolerance = 0.2 mm"
equation "BaseSupportHeight = 18 mm"
equation "buttonOD = 28 mm"
equation "ButtonTopHeight = 11 mm"
equation "ButtonTopPoleHeight = 7 mm"
equation "ButtonBottomLength = 38 mm"
equation "ButtonBottomWidth = 33.5 mm"
equation "ButtonHoleDFC = ( 43.233 / 2 ) * 1 mm"
equation "RampHeightMin = 36 mm"
equation "PowerWidth = 165 mm" comment "6.5 inch (Actual 6)"
equation "RampWidth = 40 mm"
equation "PowerLength = 155 mm" comment "6.1 (Act 5.6 inch)"
equation "PowerHeight = 100 mm"
equation "ControlBoxWidth = 100 mm"
equation "toleranceSlide = 1 mm"
equation "BoxLidButtonWallHeight = 8 mm"
equation "magnetDFE = 3.5 mm"
equation "SlideWallRemoveLength = 10 mm"
equation "SlideWallWidth = 2 mm"
equation "FiletLidRadius = 2 mm"
equation "d261 = ButtonBottomWidth"
equation "d262 = ButtonBottomLength"
equation "ButtonBottomWidthFinal = 32 mm"
equation "d264 = wallThickness"
equation "d267 = magnetOD"
equation "d269 = magnetDepth"
equation "d272 = MagnetThruHoleOD"
equation "ButtonPoleLength = 8.5 mm"
equation "ButtonPoleWidth = 5.5 mm"
equation "d290 = ButtonPoleLength"
equation "d291 = ButtonPoleWidth"
equation "d295 = ButtonTopHeight"
equation "d297 = ButtonPoleLength - PressFitTolerance"
equation "d298 = ButtonPoleWidth - PressFitTolerance"
equation "d299 = ButtonTopPoleHeight"
equation "magnetDFCWidth = 13 mm"
equation "magnetDFCLength = 15 mm"
equation "ButtonSpacing = 36.5 mm"
equation "ClearanceButton = 6.25 mm"
equation "d337 = ( ButtonSpacing * 2 ) + ClearanceButton - 3 mm - PressFitTolerance"
equation "d338 = BaseWidth"
equation "d339 = wallThickness"
equation "d341 = capsenseWidth"
equation "d342 = capsenseLength"
equation "d343 = ButtonSpacing / 2"
equation "d346 = magnetOD"
equation "d347 = magnetDFCapsense"
equation "d348 = magnetDFCapsense"
equation "d349 = magnetDFCapsense"
equation "d350 = magnetDFCapsense"
equation "d351 = -magnetDepth"
equation "d353 = MagnetThruHoleOD"
equation "d358 = ButtonSpacing / 2"
equation "d359 = capsenseWidth"
equation "d362 = CapsenseThick"
equation "d363 = wallThickness / 2"
equation "d364 = wallThickness / 2"
equation "d365 = CapsenseThick"
equation "d370 = ButtonSpacing"
equation "d372 = ( ButtonSpacing * 2 ) + ClearanceButton"
equation "d375 = boxHeight"
equation "d377 = wallThickness"
equation "d378 = boxWidth - ( 2 * wallThickness )"
equation "d379 = boxWidth"
equation "d382 = ( ButtonSpacing * 2 ) + ClearanceButton - 3 mm - 2.5 mm"
equation "d384 = BaseSupportHeight"
equation "d393 = magnetDFE"
equation "d394 = magnetDFE"
equation "d397 = magnetDFE"
equation "d398 = magnetDFE"
equation "d399 = magnetOD"
equation "d400 = -magnetDepth"
equation "d407 = -wallThickness"
equation "d413 = ButtonSpacing * 2 + ClearanceButton"
equation "d414 = boxWidth"
equation "d415 = wallThickness"
equation "d417 = buttonOD + toleranceSlide"
equation "d418 = ButtonSpacing / 2"
equation "d419 = ButtonSpacing"
equation "d422 = magnetOD"
equation "d423 = magnetDFE"
equation "d424 = magnetDFE"
equation "d425 = magnetDFE"
equation "d426 = magnetDFE"
equation "d427 = magnetDepth"
equation "d429 = ButtonBottomWidth + toleranceSlide"
equation "d430 = ButtonBottomLength + toleranceSlide"
equation "d433 = ButtonBottomWidth + toleranceSlide"
equation "d434 = ButtonBottomLength + toleranceSlide"
equation "d452 = BaseWallHeight"
equation "d455 = ButtonSpacing / 2"
equation "d456 = capsenseWidth"
equation "d457 = capsenseLength"
equation "d458 = ButtonSpacing / 2"
equation "d459 = magnetDFCapsense"
equation "d460 = magnetDFCapsense"
equation "d462 = MagnetThruHoleOD"
equation "d465 = ButtonSpacing / 2"
equation "d466 = buttonOD"
equation "d467 = ButtonSpacing / 2"
named bodies: "Button Bottom", "Button Top"
